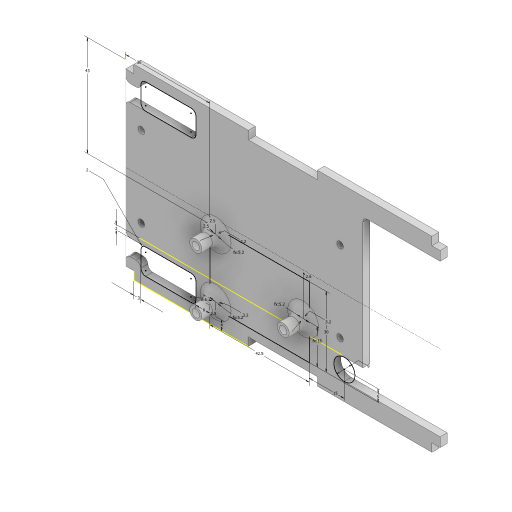
# Autodesk Inventor part: base_herelink
Saved by Autodesk Inventor 2023 (Build 270158000, 158)
## iProperties
Created: 2022-05-18
Part Number: base_herelink
Material: Generic
Document SubType Name: Modeling
Designer: Thomas
Density: 1 g/cm^3
Appearance: Default
Author: Thomas
Autodesk Inventor part; units mm, degrees
ref_plane "YZ Plane" through (0, 0, 0) normal (1, 0, 0) x (0, 1, 0)
ref_plane "XZ Plane" through (0, 0, 0) normal (0, 1, 0) x (-1, 0, 0)
ref_plane "XY Plane" through (0, 0, 0) normal (0, 0, 1) x (1, 0, 0)
sketch "Sketch1" plane through (0, 0, 0) normal (0, 0, 1) x (1, 0, 0)
  line L0 (0, 0) -> (134.5, 0)
  line L1 (134.5, 0) -> (134.5, -80)
  line L2 (134.5, -80) -> (0, -80)
  line L3 (0, -80) -> (0, 0)
  line L4 (0, 0) -> (3.5, 0)
  line L5 (3.5, 0) -> (3.5, -3.5)
  line L6 (3.5, -3.5) -> (0, -3.5)
  line L7 (0, -3.5) -> (0, 0)
  line L8 (52.5, 0) -> (82, 0)
  line L9 (82, 0) -> (82, -3.5)
  line L10 (82, -3.5) -> (52.5, -3.5)
  line L11 (52.5, -3.5) -> (52.5, 0)
  line L12 (134.5, 0) -> (131, 0)
  line L13 (131, 0) -> (131, -3.5)
  line L14 (131, -3.5) -> (134.5, -3.5)
  line L15 (134.5, -3.5) -> (134.5, 0)
  line L16 (0, -80) -> (3.5, -80)
  line L17 (3.5, -80) -> (3.5, -76.5)
  line L18 (3.5, -76.5) -> (0, -76.5)
  line L19 (0, -76.5) -> (0, -80)
  line L20 (52.5, -76.5) -> (82, -76.5)
  line L21 (82, -76.5) -> (82, -80)
  line L22 (82, -80) -> (52.5, -80)
  line L23 (52.5, -80) -> (52.5, -76.5)
  line L24 (131, -76.5) -> (134.5, -76.5)
  line L25 (134.5, -76.5) -> (134.5, -80)
  line L26 (134.5, -80) -> (131, -80)
  line L27 (131, -80) -> (131, -76.5)
  point P0 (0, -40)
  point P1 (134.5, -40)
  dimension "d0" = 134.5
  dimension "d1" = 80
  dimension "d2" = 3.5
  dimension "d3" = 3.5
  dimension "d4" = 3.5
  dimension "d5" = 3.5
  dimension "d6" = 49
  dimension "d7" = 49
  dimension "d8" = 3.5
  dimension "d9" = 3.5
  constraints: 56 end point, 14 parallel, 7 horizontal, 7 perpendicular, 5 point on line, 2 midpoint
  measures "d0" distance of L1.end L2.end
  measures "d1" distance of L0.end L1.end
  measures "d2" distance of L5.end L6.end
  measures "d3" distance of L4.end L5.end
  measures "d4" distance of L14.end L13.end
  measures "d5" distance of L13.end L12.end
  measures "d6" distance between parallel lines of L11 L5
  measures "d7" distance between parallel lines of L13 L9
  measures "d8" distance of L18.end L17.end
  measures "d9" distance of L17.end L16.end
extrude "Base Plate" add sketch "Sketch1" along normal blind 3 contours L0 L11 L10 L9 L13 L14 L1 L24 L27 L2 L21 L20 L23 L17 L18 L3 L6 L5
sketch "Sketch2" plane through (0, 0, 0) normal (0, 0, -1) x (-1, 0, 0)
  line L0 (-6, -62.145) -> (-92.46, -62.145)
  line L1 (-96.46, -58.145) -> (-96.46, -21.855)
  line L2 (-92.46, -17.855) -> (-6, -17.855)
  line L3 (-2, -21.855) -> (-2, -58.145)
  line L4 (0, -3.5) -> (0, -76.5) projected
  arc A0 (-6, -62.145) -> (-2, -58.145) centre (-6, -58.145) ccw
  arc A1 (-2, -21.855) -> (-6, -17.855) centre (-6, -21.855) ccw
  arc A2 (-96.46, -58.145) -> (-92.46, -62.145) centre (-92.46, -58.145) ccw
  arc A3 (-92.46, -17.855) -> (-96.46, -21.855) centre (-92.46, -21.855) ccw
  line L5 (-92.46, -63.145) -> (-6, -63.145)
  arc A4 (-6, -63.145) -> (-1, -58.145) centre (-6, -58.145) ccw
  line L6 (-1, -58.145) -> (-1, -21.855)
  arc A5 (-1, -21.855) -> (-6, -16.855) centre (-6, -21.855) ccw
  line L7 (-6, -16.855) -> (-92.46, -16.855)
  arc A6 (-92.46, -16.855) -> (-97.46, -21.855) centre (-92.46, -21.855) ccw
  line L8 (-97.46, -21.855) -> (-97.46, -58.145)
  arc A7 (-97.46, -58.145) -> (-92.46, -63.145) centre (-92.46, -58.145) ccw
  circle A8 centre (-6.73, -57.2) radius 1.4
  circle A9 centre (-91.73, -57.2) radius 1.4
  circle A10 centre (-6.73, -22.8) radius 1.4
  circle A11 centre (-91.73, -22.8) radius 1.4
  point P0 (0, 0)
  point P1 (-2, -62.145)
  point P2 (-96.46, -62.145)
  point P3 (-2, -17.855)
  point P4 (0, -40)
  point P5 (-2, -40)
  dimension "d12" = 44.29
  dimension "d13" = 0
  dimension "d14" = 94.46
  dimension "d15" = 2
  dimension "d16" = 4
  dimension "d17" = 1
  dimension "d18" = 2.8
  dimension "d21" = 85
  dimension "d24" = 34.4
  dimension "d27" = 4.73
  dimension "d28" = 4.945
  constraints: 16 end point, 16 point on circle, 12 centre point, 8 tangent, 6 point on line, 4 parallel, 3 equal radius, 2 horizontal, 2 midpoint, 2 perpendicular, 1 vertical, 13 other
  measures "d12" distance of point (-2, -17.855) point (-2, -62.145)
  measures "d13" vertical distance of point (0, -40) point (-2, -40)
  measures "d14" distance of point (-2, -62.145) point (-96.46, -62.145)
  measures "d15" distance between parallel lines of L4 L3
  measures "d16" radius of A0
  measures "d17" distance between parallel lines of L0 L5
  measures "d18" diameter of A8
  measures "d21" distance of A8.centre A9.centre
  measures "d24" distance of A8.centre A10.centre
  measures "d27" distance from line of A8.centre L3
  measures "d28" distance from line of A8.centre L0
extrude "CubePilot Outline" cut sketch "Sketch2" against normal blind 0.5 contours A7 L8 A6 L7 A5 L6 A4 L5
extrude "Extrusion3" cut sketch "Sketch2" against normal through all contours A8 | A9 | A10 | A11
sketch "Sketch3" plane through (0, 0, 3) normal (0, 0, 1) x (1, 0, 0)
  line L0 (36, -43) -> (78.5, -43)
  line L1 (78.5, -43) -> (78.5, -73)
  line L2 (78.5, -73) -> (36, -73)
  line L3 (36, -73) -> (36, -43)
  circle A0 centre (75.9, -58) radius 1.6
  circle A1 centre (38.5, -70.5) radius 1.6
  circle A2 centre (38.5, -45.5) radius 1.6
  circle A3 centre (93.5, -68) radius 4.5
  line L4 (8.5, -65.145) -> (28, -65.145)
  line L5 (30, -67.145) -> (30, -74)
  line L6 (28, -76) -> (8.5, -76)
  line L7 (6.5, -74) -> (6.5, -67.145)
  line L8 (3.5, -76.5) -> (3.5, -80) projected
  line L9 (3.5, -80) -> (52.5, -80) projected
  line L10 (6, -63.145) -> (92.46, -63.145) projected
  arc A4 (8.5, -65.145) -> (6.5, -67.145) centre (8.5, -67.145) ccw
  arc A5 (6.5, -74) -> (8.5, -76) centre (8.5, -74) ccw
  arc A6 (28, -76) -> (30, -74) centre (28, -74) ccw
  arc A7 (30, -67.145) -> (28, -65.145) centre (28, -67.145) ccw
  circle A8 centre (38.5, -45.5) radius 2.6
  circle A9 centre (38.5, -70.5) radius 2.6
  circle A10 centre (75.9, -58) radius 2.6
  line L11 (0, -3.5) -> (0, -76.5) projected
  line L12 (0, -40) -> (134.6587, -40) construction
  line L13 (8.5, -14.855) -> (28, -14.855)
  line L14 (30, -12.855) -> (30, -6)
  line L15 (28, -4) -> (8.5, -4)
  line L16 (6.5, -6) -> (6.5, -12.855)
  arc A11 (6.5, -12.855) -> (8.5, -14.855) centre (8.5, -12.855) ccw
  arc A12 (8.5, -4) -> (6.5, -6) centre (8.5, -6) ccw
  arc A13 (30, -6) -> (28, -4) centre (28, -6) ccw
  arc A14 (28, -14.855) -> (30, -12.855) centre (28, -12.855) ccw
  point P0 (0, 0)
  dimension "d33" = 42.5
  dimension "d34" = 30
  dimension "d35" = 43
  dimension "d36" = 36
  dimension "d37" = 3.2
  dimension "d38" = 3.2
  dimension "d39" = 3.2
  dimension "d40" = 2.5
  dimension "d41" = 2.5
  dimension "d42" = 2.5
  dimension "d43" = 2.5
  dimension "d44" = 2.6
  dimension "d45" = 15
  dimension "d46" = 9
  dimension "d47" = 5
  dimension "d48" = 15
  dimension "d49" = 3
  dimension "d50" = 4
  dimension "d51" = 2
  dimension "d52" = 6
  dimension "d53" = 2
  dimension "d54" = 5.2
  dimension "d55" = 5.2
  dimension "d56" = 5.2
  constraints: 26 end point, 16 point on circle, 15 centre point, 12 symmetric about line, 8 tangent, 4 parallel, 3 coincident, 3 equal radius, 3 horizontal, 2 perpendicular, 1 midpoint, 4 other
  measures "d33" distance of L1.end L2.end
  measures "d34" distance of L0.end L1.end
  measures "d35" distance from line of point (0, 0) L0
  measures "d36" distance from line of point (0, 0) L3
  measures "d37" diameter of A0
  measures "d38" diameter of A1
  measures "d39" diameter of A2
  measures "d40" distance from line of A2.centre L0
  measures "d41" distance from line of L3 A2.centre
  measures "d42" distance from line of L3 A1.centre
  measures "d43" distance from line of L2 A1.centre
  measures "d44" distance from line of L1 A0.centre
  measures "d45" distance from line of A0.centre L2
  measures "d46" diameter of A3
  measures "d47" distance from line of A3.centre L2
  measures "d48" distance from line of L1 A3.centre
  measures "d49" distance between parallel lines of L8 L7
  measures "d50" distance between parallel lines of L9 L6
  measures "d51" distance between parallel lines of L10 L4
  measures "d52" distance between parallel lines of L3 L5
  measures "d53" radius of A4
  measures "d54" diameter of A8
  measures "d55" diameter of A10
  measures "d56" diameter of A9
extrude "Extrusion4" add sketch "Sketch3" along normal blind 8.5 contours A8 L0 | L0 A8 L3 | L3 A8 | A10 | A9 L2 L3 | L3 A9 | L2 A9 picked at (38.4357, -43.3039) picked at (38.4357, -72.6961)
fillet "Fillet1" radius 4 3 edges at (35.9, -45.5, 3) (73.3, -58, 3) (35.9, -70.5, 3)
sketch "Sketch4" plane through (0, 0, 0) normal (0, 0, -1) x (-1, 0, 0)
  circle A0 centre (-75.9, -58) radius 1.6 projected
  circle A1 centre (-38.5, -45.5) radius 1.6 projected
  circle A2 centre (-38.5, -70.5) radius 1.6 projected
  line L0 (-41.4, -72.1743) -> (-41.4, -68.8257)
  line L1 (-41.4, -68.8257) -> (-38.5, -67.1514)
  line L2 (-38.5, -67.1514) -> (-35.6, -68.8257)
  line L3 (-35.6, -68.8257) -> (-35.6, -72.1743)
  line L4 (-35.6, -72.1743) -> (-38.5, -73.8486)
  line L5 (-38.5, -73.8486) -> (-41.4, -72.1743)
  line L6 (-38.5, -48.8486) -> (-41.4, -47.1743)
  line L7 (-41.4, -47.1743) -> (-41.4, -43.8257)
  line L8 (-41.4, -43.8257) -> (-38.5, -42.1514)
  line L9 (-38.5, -42.1514) -> (-35.6, -43.8257)
  line L10 (-35.6, -43.8257) -> (-35.6, -47.1743)
  line L11 (-35.6, -47.1743) -> (-38.5, -48.8486)
  line L12 (-75.9, -61.3486) -> (-78.8, -59.6743)
  line L13 (-78.8, -59.6743) -> (-78.8, -56.3257)
  line L14 (-78.8, -56.3257) -> (-75.9, -54.6514)
  line L15 (-75.9, -54.6514) -> (-73, -56.3257)
  line L16 (-73, -56.3257) -> (-73, -59.6743)
  line L17 (-73, -59.6743) -> (-75.9, -61.3486)
  point P0 (0, 0)
  point P1 (-35.6, -70.5)
  dimension "d60" = 5.8
  dimension "d61" = 5.8
  dimension "d62" = 5.8
  constraints: 36 end point, 3 coincident, 3 vertical, 1 midpoint, 39 other
  measures "d60" distance between parallel lines of L3 L0
  measures "d61" distance between parallel lines of L10 L7
  measures "d62" distance between parallel lines of L13 L16
extrude "Extrusion5" cut sketch "Sketch4" against normal blind 2.8 contours A0 | A1 | A2 | L0 L1 L2 L3 L4 L5 | L6 L7 L8 L9 L10 L11 | L12 L13 L14 L15 L16 L17
extrude "Extrusion6" cut sketch "Sketch3" against normal through all contours A3 | L4 A7 L5 A6 L6 A5 L7 A4 | A11 L16 A12 L15 A13 L14 A14 L13
sketch "Sketch5" plane through (0, 0, 3) normal (0, 0, 1) x (1, 0, 0)
  line L0 (103.46, -7.5) -> (132.5, -7.5)
  line L1 (134.5, -9.5) -> (134.5, -70.5)
  line L2 (132.5, -72.5) -> (101.46, -72.5)
  line L3 (101.46, -72.5) -> (101.46, -9.5)
  line L4 (131, 0) -> (82, 0) projected
  line L5 (82, -80) -> (131, -80) projected
  line L6 (134.5, -76.5) -> (134.5, -3.5) projected
  line L7 (97.46, -58.145) -> (97.46, -21.855) projected
  arc A0 (103.46, -7.5) -> (101.46, -9.5) centre (103.46, -9.5) ccw
  circle A1 centre (93.5, -68) radius 4.5 projected
  line L8 (93.5, -72.5) -> (101.46, -72.5)
  line L9 (93.5, -63.5) -> (101.46, -63.5)
  line L10 (86.46, -9.5) -> (45, -9.5) construction
  line L11 (86.46, -7) -> (45, -7)
  line L12 (45, -12) -> (86.46, -12)
  arc A2 (86.46, -12) -> (86.46, -7) centre (86.46, -9.5) ccw
  arc A3 (45, -7) -> (45, -12) centre (45, -9.5) ccw
  line L13 (30, -6) -> (30, -12.855) projected
  line L14 (82, -3.5) -> (52.5, -3.5) projected
  line L15 (132.5, -7.5) -> (134.5, -7.5)
  line L16 (132.5, -72.5) -> (134.5, -72.5)
  point P0 (0, 0)
  point P1 (65.73, -9.5)
  dimension "d67" = 7.5
  dimension "d68" = 7.5
  dimension "d69" = 0
  dimension "d70" = 4
  dimension "d71" = 2
  dimension "d74" = 12
  dimension "d75" = 5
  dimension "d76" = 15
  dimension "d77" = 15
  dimension "d78" = 6
  constraints: 24 end point, 8 point on circle, 6 tangent, 4 parallel, 3 centre point, 3 perpendicular, 3 point on line, 2 horizontal, 1 collinear, 1 midpoint
  measures "d67" distance between parallel lines of L0 L4
  measures "d68" distance between parallel lines of L5 L2
  measures "d69" distance between parallel lines of L6 L1
  measures "d70" distance between parallel lines of L7 L3
  measures "d71" radius of A0
  measures "d74" distance from line of L5 A1.centre
  measures "d75" diameter of A3
  measures "d76" distance from line of L10.start L3
  measures "d77" distance from line of L13 L10.end
  measures "d78" distance between parallel lines of L14 L10
extrude "Extrusion7" cut sketch "Sketch5" against normal through all contours L0 L15 L6 L1 L16 L2 L3 A0 | L3 L8 A1 L9
sketch "Sketch6" plane through (0, 0, 3) normal (0, 0, 1) x (1, 0, 0)
  line L0 (28, -14.855) -> (8.5, -14.855) projected
  line L1 (8.5, -14.855) -> (0, -14.855)
  line L2 (6.5, -12.855) -> (6.5, -6) projected
  line L3 (0, -3.5) -> (0, -76.5) projected
  line L4 (0, -8) -> (4.5, -8)
  line L5 (52.5, 0) -> (3.5, 0) projected
  line L6 (3.5, -3.5) -> (0, -3.5) projected
  arc A0 (8.5, -4) -> (6.5, -6) centre (8.5, -6) ccw projected
  line L7 (6.5, -6) -> (6.5, -6)
  arc A1 (4.5, -8) -> (6.5, -6) centre (4.5, -6) ccw
  line L8 (8.5, -65.145) -> (28, -65.145) projected
  line L9 (8.5, -65.145) -> (0, -65.145)
  line L10 (6.5, -74) -> (6.5, -67.145) projected
  line L11 (0, -72) -> (4.5, -72)
  line L12 (3.5, -80) -> (52.5, -80) projected
  line L13 (6.5, -67.145) -> (6.5, -74) projected
  line L14 (6.5, -74) -> (6.5, -74)
  arc A2 (6.5, -74) -> (4.5, -72) centre (4.5, -74) ccw
  arc A3 (6.5, -12.855) -> (8.5, -14.855) centre (8.5, -12.855) ccw projected
  arc A4 (6.5, -74) -> (8.5, -76) centre (8.5, -74) ccw projected
  arc A5 (8.5, -65.145) -> (6.5, -67.145) centre (8.5, -67.145) ccw projected
  point P0 (0, 0)
  point P1 (6.5, -8)
  point P2 (6.5, -72)
  dimension "d79" = 8
  dimension "d80" = 2
  dimension "d81" = 8
  dimension "d82" = 2
  constraints: 12 end point, 9 point on line, 5 tangent, 4 point on circle, 2 centre point, 2 collinear, 2 horizontal, 2 perpendicular
  measures "d79" distance between parallel lines of L4 L5
  measures "d80" radius of A1
  measures "d81" distance between parallel lines of L11 L12
  measures "d82" radius of A2
extrude "Extrusion8" cut sketch "Sketch6" against normal through all
fillet "Fillet2" radius 2 4 edges at (0, -14.855, 1.5) (0, -8, 1.5) (0, -65.145, 1.5) (0, -72, 1.5)
equation "\"d27\" = -0.5 * d21 + 0.5 * d14"
equation "\"d28\" = -0.5 * d24 + 0.5 * d12"
equation "\"d45\" = 0.5 * d34"
equation "\"d55\" = d54"
equation "\"d56\" = d54"
equation "\"d60\" = d61"
equation "\"d62\" = d61"
equation "\"d67\" = d68"
equation "\"d68\" = d74 - 0.5 * d46"
body "Solid1"
